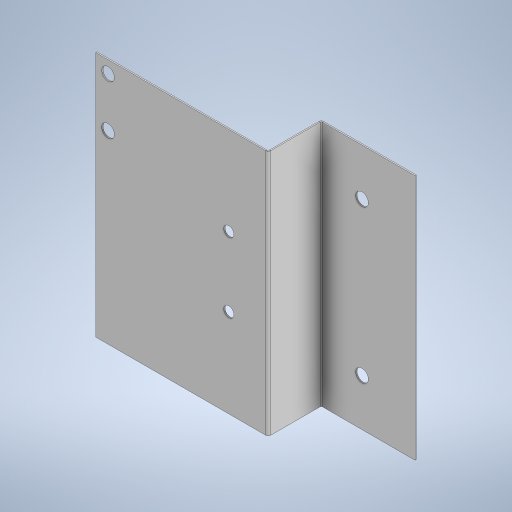
# Autodesk Inventor part: Placa Montaje
Saved by Autodesk Inventor 2023.1 (Build 271208000, 208)
## iProperties
Created: 2022-11-11
Part Number: Placa Montaje
Material: Generic
Document SubType Name: Sheet Metal
Designer: Daniel Peña
Density: 1 g/cm^3
Sheet Metal Rule: Default_mm
Appearance: Default
Author: Daniel Peña
Autodesk Inventor part; units mm, degrees
ref_plane "YZ Plane" through (0, 0, 0) normal (1, 0, 0) x (0, 1, 0)
ref_plane "XZ Plane" through (0, 0, 0) normal (0, 1, 0) x (-1, 0, 0)
ref_plane "XY Plane" through (0, 0, 0) normal (0, 0, 1) x (1, 0, 0)
sketch "Sketch1" plane through (0, 0, 0) normal (0, 0, 1) x (1, 0, 0)
  line L0 (31.1987, 43.9856) -> (69.7487, 43.9856)
  line L1 (69.7487, 43.9856) -> (69.7487, -56.0144)
  line L2 (69.7487, -56.0144) -> (31.1987, -56.0144)
  line L3 (31.1987, -56.0144) -> (31.1987, 43.9856)
  point P0 (0, 0)
  dimension "d0" = 100
  dimension "d1" = 38.55
  measures "d0" distance of L0.end L1.end
  measures "d1" distance of L1.end L2.end
extrude "Plate1" add sketch "Sketch1" along normal blind 0.5
sketch "Sketch2" plane through (31.6987, -56.0144, 0) normal (-1, 0, 0) x (0, -1, 0)
  line L0 (-100, 0) -> (0, 0)
  line L1 (0, 0) -> (0, 22)
  line L2 (0, 22) -> (-100, 22)
  line L3 (-100, 22) -> (-100, 0)
  constraints: 6 end point, 1 horizontal, 1 perpendicular, 1 vertical
edge flange "Flange1" height 22 angle 90 thickness 0.5 bend radius 0.5 thickness toward (-1, 0, 0) relief straight relief width 0.5 relief depth 0.25 edges at (31.1987, -6.0144, 0.5) wall of the first edge with corners at (31.6987, 43.9856, 0) (31.6987, -56.0144, 0) (31.6987, -56.0144, 22) (31.6987, 43.9856, 22)
bend "Bend1"
corner "Corner1"
sketch "Sketch3" plane through (31.6987, 43.9856, 21.5) normal (0, 0, 1) x (1, 0, 0)
  line L0 (0, -100) -> (0, 0)
  line L1 (0, 0) -> (-70, 0)
  line L2 (-70, 0) -> (-70, -100)
  line L3 (-70, -100) -> (0, -100)
  constraints: 6 end point, 1 horizontal, 1 perpendicular, 1 vertical
edge flange "Flange2" height 70 angle 90 thickness 0.5 bend radius 0.5 thickness toward (0, 0, 1) relief straight relief width 0.5 relief depth 0.25 edges at (31.1987, -6.0144, 22) wall of the first edge with corners at (31.6987, -56.0144, 21.5) (31.6987, 43.9856, 21.5) (-38.3013, 43.9856, 21.5) (-38.3013, -56.0144, 21.5)
bend "Bend2"
corner "Corner2"
sketch "Sketch4" plane through (0, 0, 0.5) normal (0, 0, 1) x (1, 0, 0)
  line L0 (48.2487, 25.2184) -> (48.2487, -36.8148) construction
  line L1 (32.1987, 43.9856) -> (69.7487, 43.9856) projected
  line L2 (69.7487, -56.0144) -> (32.1987, -56.0144) projected
  line L3 (69.7487, 43.9856) -> (69.7487, -56.0144) projected
  point P0 (0, 0)
  point P1 (48.2487, 24.9856)
  point P2 (48.2487, -37.0144)
  dimension "d23" = 19
  dimension "d24" = 62
  dimension "d25" = 19
  dimension "d26" = 21.5
  constraints: 2 end point, 2 point on line, 1 vertical
  measures "d23" distance from line of L1 point (48.249, 24.986)
  measures "d24" distance of point (48.249, 24.986) point (48.249, -37.014)
  measures "d25" distance from line of L2 point (48.249, -37.014)
  measures "d26" distance from line of L3 point (48.249, -37.014)
hole "Hole1" at (48.2487, 24.9856, 0.5) at (48.2487, -37.0144, 0.5) direction (0, 0, -1) diameter 5.1 end through all
sketch "Sketch5" plane through (-38.3013, -56.0144, 22) normal (0, 0, 1) x (1, 0, 0)
  line L0 (54, 64.1) -> (54, 35.9) construction
  line L1 (0, 100) -> (69, 100) projected
  line L2 (69, 0) -> (0, 0) projected
  line L3 (69, 0) -> (69, 100) projected
  point P0 (38.3013, 56.0144)
  dimension "d34" = 28.2
  dimension "d35" = 35.9
  dimension "d36" = 35.9
  dimension "d37" = 15
  constraints: 2 end point, 1 vertical
  measures "d34" distance of L0.end L0.start
  measures "d35" distance from line of L1 L0.start
  measures "d36" distance from line of L2 L0.end
  measures "d37" distance between parallel lines of L3 L0
hole "Hole2" at (15.6987, 8.0856, 22) at (15.6987, -20.1144, 22) direction (0, 0, -1) diameter 4.1 end through all
sketch "Sketch6" plane through (-38.3013, -56.0144, 22) normal (0, 0, 1) x (1, 0, 0)
  line L0 (5, 95) -> (5, 75) construction
  line L1 (0, 100) -> (69, 100) projected
  line L2 (0, 0) -> (0, 100) projected
  point P0 (38.3013, 56.0144)
  dimension "d45" = 20
  dimension "d46" = 5
  dimension "d47" = 5
  constraints: 2 end point, 1 vertical
  measures "d45" distance of L0.start L0.end
  measures "d46" distance from line of L1 L0.start
  measures "d47" distance from line of L2 L0.start
hole "Hole3" at (-33.3013, 38.9856, 22) at (-33.3013, 18.9856, 22) direction (0, 0, -1) diameter 5.1 end through all
equation "\"d23\" = d25"
equation "\"d32\" = Thickness"
equation "\"d35\" = d36"
equation "\"d2\" = Thickness"
equation "\"d3\" = BendReliefWidth"
equation "\"d4\" = BendReliefDepth"
equation "\"d5\" = MinimumRemnant"
equation "\"d6\" = TransitionRadius"
equation "\"d9\" = BendRadius"
equation "\"d10\" = CornerReliefSize"
equation "\"d11\" = GapSize"
equation "\"d12\" = JacobiRadiusSize"
equation "\"d13\" = BendReliefWidth"
equation "\"d14\" = BendReliefDepth"
equation "\"d15\" = MinimumRemnant"
equation "\"d16\" = TransitionRadius"
equation "\"d19\" = BendRadius"
equation "\"d20\" = CornerReliefSize"
equation "\"d21\" = GapSize"
equation "\"d22\" = JacobiRadiusSize"
equation "\"BendRadius\" = Thickness"
equation "\"BendReliefWidth\" = Thickness"
equation "\"BendReliefDepth\" = 0.5 * Thickness"
equation "\"CornerReliefSize\" = 4 * Thickness"
equation "\"MinimumRemnant\" = 2 * Thickness"
equation "\"TransitionRadius\" = BendRadius"
equation "\"JacobiRadiusSize\" = BendRadius"
equation "\"GapSize\" = Thickness"
equation "\"Thickness\" = 0.5"
body "Solid1"
